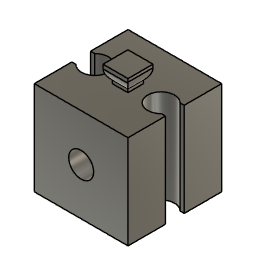
ReedSensorHalter v1 (Autodesk Fusion 360 design; units mm, degrees)
Autodesk Fusion 360 part; units mm, degrees
sketch "Skizze1" plane through (0, 0, 0) normal (0, 1, 0) x (1, 0, 0)
  line L0 (0, 0) -> (15, 0)
  line L1 (15, 0) -> (15, -15)
  line L2 (15, -15) -> (0, -15)
  line L3 (0, -15) -> (0, 0)
  dimension "d1" = 15
  dimension "d2" = 15
  constraint horizontal L0
  constraint vertical L1
  constraint horizontal L2
  constraint vertical L3
  constraint coincident L0.start L3.end
  measures "d1" distance of L0.start L0.end
  measures "d2" distance of L0.start L2.end
extrude "Extrusion1" add sketch "Skizze1" along normal blind 15
sketch "Skizze2" plane through (0, 0, 15) normal (0, 0, 1) x (-1, 0, 0)
  line L0 (0, 0) -> (-15, 0)
  line L1 (-15, 0) -> (-15, -15)
  line L2 (0, -15) -> (0, 0)
  line L3 (0, -6) -> (0, -7.5)
  line L4 (-1, -6) -> (0, -6)
  line L5 (-1, -7.5) -> (-1, -6)
  line L6 (0, -7.5) -> (0, -9)
  line L7 (-1, -7.5) -> (-1, -6)
  line L8 (0, -9) -> (-1, -9)
  line L9 (-1, -9) -> (-1, -7.5)
  circle A0 centre (-2.2, -7.5) radius 2.15
  line L10 (0, -9) -> (-1, -9)
  line L11 (-2.2, -7.5) -> (0, -7.5)
  line L12 (-1, -9) -> (-1, -7.5)
  circle A1 centre (-2.2, -7.5) radius 2.15
  line L13 (0, -7.5) -> (0, -9)
  line L14 (0, 0) -> (0, -15)
  line L15 (-2.2, -7.5) -> (0, -7.5)
  circle A2 centre (-2.2, -7.5) radius 2.15
  line L16 (0, -6) -> (0, -7.5)
  line L17 (-1, -6) -> (0, -6)
  line L18 (0, -15) -> (0, 0)
  circle A3 centre (-2.2, -7.5) radius 2.15
  circle A4 centre (-12.8, -7.5) radius 2.15
  circle A5 centre (-12.8, -7.5) radius 2.15
  line L19 (-12.8, -7.5) -> (-15, -7.5)
  line L20 (-14, -6) -> (-14, -7.5)
  line L21 (-15, -6) -> (-14, -6)
  line L22 (-14, -7.5) -> (-14, -9)
  circle A6 centre (-12.8, -7.5) radius 2.15
  line L23 (-15, -7.5) -> (-15, -6)
  circle A7 centre (-12.8, -7.5) radius 2.15
  line L24 (-15, -9) -> (-15, -7.5)
  line L25 (-14, -6) -> (-14, -7.5)
  line L26 (-14, -9) -> (-15, -9)
  line L27 (-14, -9) -> (-15, -9)
  line L28 (-15, -9) -> (-15, -7.5)
  line L29 (-15, -6) -> (-14, -6)
  line L30 (-15, -7.5) -> (-15, -6)
  line L31 (-12.8, -7.5) -> (-15, -7.5)
  line L32 (-14, -7.5) -> (-14, -9)
  line L33 (-5.5, -9.5) -> (-9.5, -9.5)
  line L34 (-9.5, -9.5) -> (-9.5, -5.5)
  line L35 (-9.5, -5.5) -> (-5.5, -5.5)
  line L36 (-5.5, -5.5) -> (-5.5, -9.5)
  point P0 (-15, -15)
  point P1 (0, -15)
  point P2 (0, -15)
  point P3 (0, -15)
  point P4 (0, 0)
  point P5 (0, 0)
  point P6 (-15, 0)
  point P7 (-15, 0)
  point P8 (-15, 0)
  point P9 (-15, 0)
  point P10 (-15, 0)
  point P11 (-15, 0)
  point P12 (-15, 0)
  dimension "d18" = 1.5
  dimension "d19" = 1
  dimension "d20" = 1.5
  dimension "d21" = 1.5
  dimension "d22" = 1
  dimension "d23" = 1.5
  dimension "d24" = 1.5
  dimension "d25" = 1
  dimension "d26" = 1.5
  dimension "d27" = 1.5
  dimension "d28" = 1
  dimension "d29" = 1.5
  dimension "d30" = 15
  dimension "d43" = 1.5
  dimension "d44" = 1
  dimension "d45" = 1.5
  dimension "d46" = 1.5
  dimension "d47" = 1
  dimension "d48" = 1.5
  dimension "d49" = 1.5
  dimension "d50" = 1
  dimension "d51" = 1.5
  dimension "d52" = 1.5
  dimension "d53" = 1
  dimension "d54" = 1.5
  dimension "d60" = 4
  dimension "d61" = 4
  constraint coincident A0.centre L11.start
  constraint perpendicular L13 L15
  constraint perpendicular L10 L13
  constraint coincident L5.start L15
  constraint perpendicular L12 L15
  constraint perpendicular L5 L15
  constraint perpendicular L4 L5
  constraint coincident L3.end L13
  constraint perpendicular L6 L11
  constraint perpendicular L6 L8
  constraint coincident L5.start L11
  constraint perpendicular L9 L11
  constraint perpendicular L7 L11
  constraint perpendicular L7 L17
  constraint coincident L3.end L6
  constraint coincident A4.centre A5.centre
  constraint perpendicular L23 L31
  constraint perpendicular L21 L23
  constraint coincident L20.end L31
  constraint perpendicular L20 L31
  constraint perpendicular L22 L31
  constraint perpendicular L22 L27
  constraint coincident L19.end L23
  constraint perpendicular L19 L30
  constraint perpendicular L29 L30
  constraint coincident L20.end L19
  constraint perpendicular L19 L25
  constraint perpendicular L19 L32
  constraint perpendicular L26 L32
  constraint coincident L19.end L30
  constraint horizontal L33
  constraint vertical L34
  constraint horizontal L35
  constraint vertical L36
  measures "d18" distance of L6.end L3.end
  measures "d19" distance of L6.end L8.end
  measures "d20" distance of L8.end L5.start
  measures "d21" distance of L5.start L4.start
  measures "d22" distance of L4.start L3.start
  measures "d23" distance of L3.end L3.start
  measures "d24" distance of L3.end L6.end
  measures "d25" distance of L8.end L6.end
  measures "d26" distance of L8.end L5.start
  measures "d27" distance of L4.start L5.start
  measures "d28" distance of L4.start L3.start
  measures "d29" distance of L3.end L3.start
  measures "d30" distance of P5 P3
  measures "d43" distance of L21.start L19.end
  measures "d44" distance of L20.start L21.start
  measures "d45" distance of L20.start L20.end
  measures "d46" distance of L20.end L22.end
  measures "d47" distance of L24.start L22.end
  measures "d48" distance of L19.end L24.start
  measures "d49" distance of L19.end L21.start
  measures "d50" distance of L21.start L20.start
  measures "d51" distance of L20.end L20.start
  measures "d52" distance of L22.end L20.end
  measures "d53" distance of L22.end L24.start
  measures "d54" distance of L19.end L24.start
  measures "d60" distance of L33.start L33.end
  measures "d61" distance of L33.start L35.end
extrude "Extrusion2" cut sketch "Skizze2" against normal blind 15 contours L1 A4 A5 L19 L21 A6 L23 A7 L29 L30 L31 | L1 A4 A5 L19 A6 A7 L24 L26 L27 L28 L31 | A4 A5 L19 L20 L21 A6 A7 L25 L29 L31 | A4 A5 L20 L21 L22 A6 A7 L25 L26 L27 L29 L32 | A4 A5 L19 L22 A6 A7 L26 L27 L31 L32 | L2 L6 L8 A0 L10 L11 A1 L13 L14 L15 A2 L18 A3 | L2 L3 L4 A0 L11 A1 L14 L15 A2 L16 L17 L18 A3 | L4 L5 L7 L8 L9 A0 L10 L12 A1 A2 L17 A3 | L8 L9 A0 L10 L11 L12 A1 L15 A2 A3 | L4 L5 L7 A0 L11 A1 L15 A2 L17 A3
extrude "Extrusion4" add sketch "Skizze2" along normal blind 2.7 contours L33 L34 L35 L36
sketch "Skizze4" plane through (0, 5.5, 0) normal (0, -1, 0) x (1, 0, 0)
  line L0 (5.5, 15) -> (9.5, 15)
  line L1 (9.5, 15) -> (9.5, 17.7)
  line L2 (9.5, 17.7) -> (5.5, 17.7)
  line L3 (5.5, 17.7) -> (5.5, 15)
  line L4 (9.5, 17.7) -> (5.5, 17.7)
  line L5 (8.739, 15.54) -> (8.739, 15)
  line L6 (5.5, 15) -> (6.261, 15)
  line L7 (9.5, 17.7) -> (9.5, 15)
  arc A0 (8.739, 15.54) -> (9.5, 17.2) centre (7.309, 17.2) ccw
  line L8 (7.489, 15.54) -> (7.489, 17.204)
  line L9 (9.5, 15) -> (9.5, 17.7)
  line L10 (6.239, 15.54) -> (8.739, 15.54)
  line L11 (9.5, 17.7) -> (5.5, 17.7)
  line L12 (6.239, 15) -> (6.239, 15.54)
  line L13 (9.5, 15) -> (9.5, 17.7)
  line L14 (9.5, 15) -> (8.739, 15)
  line L15 (9.5, 17.7) -> (5.5, 17.7)
  line L16 (5.5, 17.7) -> (9.5, 17.7)
  line L17 (5.5, 15) -> (5.5, 17.7)
  line L18 (9.5, 15) -> (5.5, 15)
  line L19 (6.239, 15.54) -> (7.489, 15.54)
  arc A1 (5.5, 17.2) -> (6.239, 15.54) centre (7.558, 17.1217) ccw
  line L20 (5.5, 15) -> (9.5, 15)
  line L21 (5.5, 17.2) -> (9.5, 17.2)
  line L22 (5.5, 17.7) -> (5.5, 15)
  line L23 (8.739, 15) -> (6.239, 15)
  line L24 (5.5, 17.7) -> (5.5, 15)
  line L25 (9.5, 17.2) -> (9.5, 17.7)
  line L26 (5.5, 17.7) -> (5.5, 17.2)
  line L27 (5.5, 15) -> (9.5, 15)
  dimension "d64" = 0.761
  dimension "d65" = 0.761
  dimension "d66" = 2.5
  dimension "d67" = 0.54
  dimension "d68" = 1.25
  dimension "d69" = 1.664
  dimension "d70" = 4
  dimension "d71" = 0.5
  constraint horizontal L16
  constraint vertical L7
  constraint horizontal L18
  constraint vertical L17
  constraint coincident L0.end L9
  constraint coincident L2.end L3.start
  constraint coincident L0.start L3.end
  constraint perpendicular L6 L17
  constraint coincident L5.end L18
  constraint horizontal L23
  constraint vertical L12
  constraint horizontal L10
  constraint vertical L5
  constraint midpoint L8.start L10
  constraint perpendicular L8 L19
  constraint horizontal L11
  constraint vertical L26
  constraint horizontal L21
  constraint vertical L25
  constraint coincident A1.start L17
  constraint coincident L1.end L2.start
  constraint tangent A0 L25
  measures "d64" distance of L6.end L0.start
  measures "d65" distance of L5.end L0.end
  measures "d66" distance of L5.end L12.start
  measures "d67" distance of L5.start L5.end
  measures "d68" distance of L8.start L10.start
  measures "d69" distance of L8.start L8.end
  measures "d70" distance of A1.start A0.end
  measures "d71" distance of L2.end A1.start
extrude "Extrusion5" cut sketch "Skizze4" against normal blind 4 contours L0 L3 L6 L12 L17 L18 A1 L20 L22 L24 L27 | L0 L1 L5 L7 A0 L9 L13 L14 L18 L20 L27
sketch "Skizze5" plane through (9.5, 0, 0) normal (1, 0, 0) x (0, 1, 0)
  line L0 (5.5, 17.2) -> (9.5, 17.2)
  line L1 (9.5, 17.2) -> (9.5, 17.7)
  line L2 (9.5, 17.7) -> (5.5, 17.7)
  line L3 (5.5, 17.7) -> (5.5, 17.2)
  line L4 (9.5, 17.7) -> (5.5, 17.7)
  line L5 (8.739, 15.54) -> (8.739, 15)
  line L6 (5.5, 15) -> (6.261, 15)
  line L7 (9.5, 17.7) -> (9.5, 15)
  arc A0 (8.739, 15.54) -> (9.5, 17.2) centre (7.309, 17.2) ccw
  line L8 (7.489, 15.54) -> (7.489, 17.204)
  line L9 (9.5, 15) -> (9.5, 17.7)
  line L10 (6.239, 15.54) -> (8.739, 15.54)
  line L11 (9.5, 17.7) -> (5.5, 17.7)
  line L12 (6.239, 15) -> (6.239, 15.54)
  line L13 (9.5, 15) -> (9.5, 17.7)
  line L14 (9.5, 15) -> (8.739, 15)
  line L15 (9.5, 17.7) -> (5.5, 17.7)
  line L16 (5.5, 17.7) -> (9.5, 17.7)
  line L17 (5.5, 15) -> (5.5, 17.7)
  line L18 (9.5, 15) -> (5.5, 15)
  line L19 (6.239, 15.54) -> (7.489, 15.54)
  arc A1 (5.5, 17.2) -> (6.239, 15.54) centre (7.558, 17.1217) ccw
  line L20 (5.5, 15) -> (9.5, 15)
  line L21 (5.5, 17.2) -> (9.5, 17.2)
  line L22 (5.5, 17.7) -> (5.5, 15)
  line L23 (8.739, 15) -> (6.239, 15)
  line L24 (5.5, 17.7) -> (5.5, 15)
  line L25 (9.5, 17.2) -> (9.5, 17.7)
  line L26 (5.5, 17.7) -> (5.5, 17.2)
  line L27 (5.5, 15) -> (9.5, 15)
  dimension "d74" = 0.761
  dimension "d75" = 0.761
  dimension "d76" = 2.5
  dimension "d77" = 0.54
  dimension "d78" = 1.25
  dimension "d79" = 1.664
  dimension "d80" = 4
  dimension "d81" = 0.5
  constraint horizontal L16
  constraint vertical L7
  constraint horizontal L18
  constraint vertical L17
  constraint coincident L7.end L9
  constraint coincident L2.end L3.start
  constraint coincident L6.start L17.start
  constraint perpendicular L6 L17
  constraint coincident L5.end L18
  constraint horizontal L23
  constraint vertical L12
  constraint horizontal L10
  constraint vertical L5
  constraint midpoint L8.start L10
  constraint perpendicular L8 L19
  constraint horizontal L11
  constraint vertical L26
  constraint horizontal L21
  constraint vertical L25
  constraint coincident L0.start L17
  constraint coincident L1.end L2.start
  constraint tangent A0 L25
  measures "d74" distance of L6.end L6.start
  measures "d75" distance of L5.end L7.end
  measures "d76" distance of L5.end L12.start
  measures "d77" distance of L5.start L5.end
  measures "d78" distance of L8.start L10.start
  measures "d79" distance of L8.start L8.end
  measures "d80" distance of L0.start L0.end
  measures "d81" distance of L2.end L0.start
extrude "Extrusion6" cut sketch "Skizze5" against normal blind 4 contours L6 L12 L17 L18 A1 L20 L22 L24 L27 | L5 L7 A0 L9 L13 L14 L18 L20 L27
sketch "Skizze3" plane through (0, 0, 0) normal (0, -1, 0) x (1, 0, 0)
  line L0 (15, 15) -> (0, 15)
  line L1 (0, 15) -> (0, 0)
  line L2 (0, 0) -> (15, 0)
  line L3 (15, 0) -> (15, 15)
  circle A0 centre (7.5, 7.5) radius 2
  dimension "d57" = 4
  measures "d57" diameter of A0
extrude "Extrusion3" cut sketch "Skizze3" against normal blind 15 contours A0
